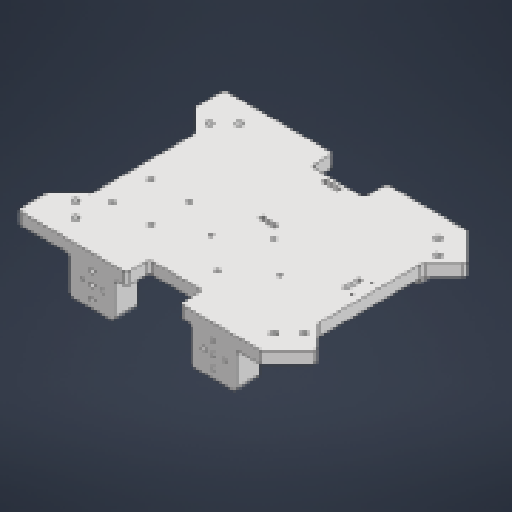
# Autodesk Inventor part: electronics panel
Saved by Autodesk Inventor 2023 (Build 270158000, 158)
## iProperties
Created: 2023-01-16
Part Number: electronics panel
Material: Generic
Document SubType Name: Modeling
Designer: Michael
Density: 1 g/cm^3
Appearance: Default
Author: Michael
Autodesk Inventor part; units mm, degrees
ref_plane "YZ Plane" through (0, 0, 0) normal (1, 0, 0) x (0, 1, 0)
ref_plane "XZ Plane" through (0, 0, 0) normal (0, 1, 0) x (-1, 0, 0)
ref_plane "XY Plane" through (0, 0, 0) normal (0, 0, 1) x (1, 0, 0)
sketch "Sketch2" plane through (0, 0, 0) normal (0, 1, 0) x (-1, 0, 0)
  line L0 (0, 0) -> (177.8, 0)
  line L1 (177.8, 0) -> (177.8, -127)
  line L2 (177.8, -127) -> (0, -127)
  line L3 (0, -127) -> (0, 0)
  line L4 (155.3506, 0) -> (177.8, -22.4519) projected
  line L5 (177.8, -104.5481) -> (155.3506, -127) projected
  line L6 (0, -22.4519) -> (22.4494, 0) projected
  line L7 (22.4494, -127) -> (0, -104.5481) projected
  line L8 (155.3506, 0) -> (173.3121, 17.9595)
  line L9 (173.3121, 17.9595) -> (195.7615, -4.4923)
  line L10 (195.7615, -4.4923) -> (177.8, -22.4519)
  line L11 (177.8, -63.5) -> (0, -63.5)
  line L12 (88.9, -127) -> (88.9, 0)
  line L13 (155.3506, -127) -> (177.8, -104.5481)
  line L14 (155.3506, -127) -> (173.3121, -144.9595)
  line L15 (173.3121, -144.9595) -> (195.7615, -122.5077)
  line L16 (195.7615, -122.5077) -> (177.8, -104.5481)
  line L17 (22.4494, 0) -> (0, -22.4519)
  line L18 (0, -104.5481) -> (22.4494, -127)
  line L19 (22.4494, 0) -> (4.4879, 17.9595)
  line L20 (4.4879, 17.9595) -> (-17.9615, -4.4923)
  line L21 (-17.9615, -4.4923) -> (0, -22.4519)
  line L22 (4.4879, -144.9595) -> (-17.9615, -122.5077)
  line L23 (22.4494, -127) -> (4.4879, -144.9595)
  line L24 (-17.9615, -122.5077) -> (0, -104.5481)
  line L25 (-17.9615, -122.5077) -> (-17.9615, -144.9595)
  line L26 (-17.9615, -144.9595) -> (4.4879, -144.9595)
  line L27 (173.3121, -144.9595) -> (195.7615, -144.9595)
  line L28 (195.7615, -144.9595) -> (195.7615, -122.5077)
  line L29 (195.7615, -4.4923) -> (195.7615, 17.9595)
  line L30 (195.7615, 17.9595) -> (173.3121, 17.9595)
  line L31 (-17.9615, -4.4923) -> (-17.9615, 17.9595)
  line L32 (4.4879, 17.9595) -> (-17.9615, 17.9595)
  line L33 (4.4879, -144.9595) -> (42.5879, -144.9595)
  line L34 (42.5879, -144.9595) -> (42.5879, -127)
  line L35 (173.3121, -144.9595) -> (135.2121, -144.9595)
  line L36 (135.2121, -144.9595) -> (135.2121, -127)
  line L37 (4.4879, 17.9595) -> (42.5879, 17.9595)
  line L38 (42.5879, 17.9595) -> (42.5879, 0)
  line L39 (173.3121, 17.9595) -> (135.2121, 17.9595)
  line L40 (135.2121, 17.9595) -> (135.2121, 0)
  circle A0 centre (178.6987, -10.7776) radius 2.4765 projected
  circle A1 centre (167.025, 0.8974) radius 2.4765 projected
  circle A2 centre (10.775, 0.8974) radius 2.4765 projected
  circle A3 centre (-0.8987, -10.7776) radius 2.4765 projected
  circle A4 centre (10.775, -127.8974) radius 2.4765 projected
  circle A5 centre (-0.8987, -116.2224) radius 2.4765 projected
  circle A6 centre (178.6987, -116.2224) radius 2.4765 projected
  circle A7 centre (167.025, -127.8974) radius 2.4765 projected
  dimension "d0" = 177.8
  dimension "d1" = 127
  dimension "d30" = 25.4
  dimension "d80" = 38.1
  constraints: 74 end point, 12 symmetric about line, 8 perpendicular, 5 point on line, 4 midpoint, 2 horizontal, 2 parallel
  measures "d0" distance of L1.end L2.end
  measures "d1" distance of L0.end L1.end
  measures "d30" distance of L4.start L8.end
  measures "d80" distance of L23.end L33.end
extrude "Extrusion8" add sketch "Sketch2" against normal blind 9.525 contours L19 L37 L38 L0 | L6 L3 A3 L0 A2 | L0 L12 L11 L3 L6 | L0 A2 L3 A3 L21 L20 L19 | L0 L4 L1 L11 L12 | L11 L12 L2 L7 L3 | L40 L39 L8 L0 | L11 L1 L5 L2 L12 | L7 L2 A4 L3 A5 | L3 A5 L2 A4 L23 L22 L24 | L8 L9 L10 L1 A0 L0 A1 | L0 A1 L1 A0 L4 | L2 L34 L33 L23 | L30 L29 L9 | L16 L15 L14 L2 A7 L1 A6 | L1 A6 L2 A7 L5 | L2 L14 L35 L36 | L28 L27 L15
sketch "Sketch8" plane through (0, 0, 0) normal (0, 1, 0) x (1, 0, 0)
  line L0 (-42.5879, 127) -> (-135.2121, 127) projected
  line L1 (0, 22.4519) -> (0, 104.5481) projected
  line L2 (-135.2121, 0) -> (-42.5879, 0) projected
  line L3 (-177.8, 104.5481) -> (-177.8, 22.4519) projected
  line L4 (-145.2802, 116.9307) -> (-173.3121, 144.9595) projected
  line L5 (-195.7615, 122.5077) -> (-177.8, 104.5481) projected
  line L6 (-177.8, 22.4519) -> (-195.7615, 4.4923) projected
  line L7 (-173.3121, -17.9595) -> (-145.2802, 10.0693) projected
  line L8 (-32.5198, 10.0693) -> (-4.4879, -17.9595) projected
  line L9 (17.9615, 4.4923) -> (0, 22.4519) projected
  line L10 (0, 104.5481) -> (17.9615, 122.5077) projected
  line L11 (-4.4879, 144.9595) -> (-32.5198, 116.9307) projected
  line L12 (-135.2121, 127) -> (-129.9506, 127)
  line L13 (-173.3121, 144.9595) -> (-135.2121, 144.9595)
  line L14 (-135.2121, 144.9595) -> (-135.2121, 127)
  line L15 (-42.5879, 127) -> (-135.2121, 127) projected
  line L16 (-135.2121, 127) -> (-109.8121, 127)
  line L17 (-109.8121, 127) -> (-109.8121, 144.9595)
  line L18 (-109.8121, 144.9595) -> (-135.2121, 144.9595)
  line L19 (-135.2121, 144.9595) -> (-135.2121, 127)
  line L20 (-42.5879, 0) -> (-135.2121, 0) projected
  line L21 (-88.9, 0) -> (-88.9, 127)
  line L22 (0, 104.5481) -> (0, 22.4519) projected
  line L23 (0, 63.5) -> (-177.8, 63.5)
  line L24 (-135.2121, 0) -> (-173.3121, -17.9595)
  line L25 (-135.2121, 0) -> (-129.9506, 0)
  line L26 (-173.3121, -17.9595) -> (-135.2121, -17.9595)
  line L27 (-135.2121, -17.9595) -> (-135.2121, 0)
  line L28 (-135.2121, 0) -> (-109.8121, 0)
  line L29 (-109.8121, 0) -> (-109.8121, -17.9595)
  line L30 (-109.8121, -17.9595) -> (-135.2121, -17.9595)
  line L31 (-135.2121, -17.9595) -> (-135.2121, 0)
  line L32 (-42.5879, 0) -> (-135.2121, 0)
  line L33 (-42.5879, 127) -> (-4.4879, 144.9595)
  line L34 (-4.4879, -17.9595) -> (-42.5879, 0)
  line L35 (-42.5879, 127) -> (-47.8494, 127)
  line L36 (-4.4879, 144.9595) -> (-42.5879, 144.9595)
  line L37 (-42.5879, 144.9595) -> (-42.5879, 127)
  line L38 (-67.9879, 127) -> (-67.9879, 144.9595)
  line L39 (-67.9879, 144.9595) -> (-42.5879, 144.9595)
  line L40 (-42.5879, 0) -> (-47.8494, 0)
  line L41 (-67.9879, 0) -> (-67.9879, -17.9595)
  line L42 (-42.5879, -17.9595) -> (-42.5879, 0)
  line L43 (-67.9879, -17.9595) -> (-42.5879, -17.9595)
  line L44 (-4.4879, -17.9595) -> (-42.5879, -17.9595)
  point P0 (0, 0)
  point P1 (-109.8121, 127)
  point P2 (-109.8121, 0)
  point P3 (-22.4494, -17.9595)
  point P4 (-67.9879, 0)
  point P5 (-22.4494, 144.9595)
  point P6 (-67.9879, 127)
  dimension "d54" = 25.4
  dimension "d56" = 0
  constraints: 60 end point, 17 symmetric about line, 4 midpoint, 3 horizontal, 2 parallel, 2 perpendicular
  measures "d54" distance of L18.end L17.end
  measures "d56" distance between parallel lines of L18 L13
extrude "Extrusion10" add sketch "Sketch8" against normal blind 9.525
sketch "Sketch10" plane through (0, -9.525, 0) normal (0, -1, 0) x (1, 0, 0)
  line L0 (-23.5379, -144.9595) -> (-23.5379, -127)
  line L1 (-109.8121, -127) -> (-67.9879, -127) projected
  line L2 (-67.9879, 0) -> (-109.8121, 0) projected
  line L3 (0, -104.5481) -> (0, -22.4519) projected
  line L4 (-177.8, -22.4519) -> (-177.8, -104.5481) projected
  line L5 (0, -63.5) -> (-177.8, -63.5)
  line L6 (-177.8, -104.5481) -> (-177.8, -22.4519) projected
  line L7 (-67.9879, -127) -> (-109.8121, -127) projected
  line L8 (-88.9, -127) -> (-88.9, 0)
  line L9 (-23.5379, -127) -> (-58.4629, -127)
  line L10 (-58.4629, -127) -> (-58.4629, -144.9595)
  line L11 (-58.4629, -144.9595) -> (-23.5379, -144.9595)
  line L12 (-23.5379, -144.9595) -> (-23.5379, -127)
  line L13 (-154.2621, -127) -> (-119.3371, -127)
  line L14 (-119.3371, -127) -> (-119.3371, -144.9595)
  line L15 (-119.3371, -144.9595) -> (-154.2621, -144.9595)
  line L16 (-154.2621, -144.9595) -> (-154.2621, -127)
  line L17 (-23.5379, 17.9595) -> (-23.5379, 0)
  line L18 (-23.5379, 0) -> (-58.4629, 0)
  line L19 (-58.4629, 0) -> (-58.4629, 17.9595)
  line L20 (-58.4629, 17.9595) -> (-23.5379, 17.9595)
  line L21 (-119.3371, 0) -> (-119.3371, 17.9595)
  line L22 (-154.2621, 0) -> (-119.3371, 0)
  line L23 (-154.2621, 17.9595) -> (-154.2621, 0)
  line L24 (-119.3371, 17.9595) -> (-154.2621, 17.9595)
  point P0 (0, 0)
  point P1 (-67.9879, -144.9595)
  point P2 (-109.8121, -144.9595)
  point P3 (-42.5879, -127)
  point P4 (-135.2121, -127)
  point P5 (-42.5879, 0)
  point P6 (-135.2121, 0)
  dimension "d81" = 34.925
  constraints: 38 end point, 14 symmetric about line, 4 midpoint, 2 parallel, 1 horizontal, 1 perpendicular
  measures "d81" distance of L11.end L10.end
extrude "Extrusion11" add sketch "Sketch10" along normal blind 28.575
sketch "Sketch13" plane through (-109.8121, 0, -144.9595) normal (0, 0, -1) x (-1, 0, 0)
  line L0 (34.986, -21.615) -> (18.9865, -21.615)
  line L1 (26.9862, -31.115) -> (26.9862, -12.115)
  line L2 (44.45, -34.925) -> (0, -34.925) projected
  line L3 (0, 0) -> (0, -9.525) projected
  line L4 (-41.8241, -9.525) -> (0, -9.525) projected
  line L5 (-20.9121, -9.525) -> (-20.9121, -25.2345)
  line L6 (-76.8101, -21.615) -> (-60.8106, -21.615)
  line L7 (-68.8104, -31.115) -> (-68.8104, -12.115)
  line L8 (9.525, -9.525) -> (9.525, -38.1) projected
  point P0 (-109.8121, 0)
  point P1 (26.9862, -21.615)
  point P2 (0, -34.925)
  point P3 (-82.1012, -6.35)
  point P4 (-68.8104, -21.615)
  point P5 (-67.2241, -9.525)
  dimension "d66" = 15.9995
  dimension "d67" = 19
  dimension "d68" = 3.81
  dimension "d83" = 9.4615
  constraints: 10 end point, 9 symmetric about line, 8 coincident, 2 midpoint, 2 vertical, 1 horizontal, 3 other
  measures "d66" distance of L0.start L0.end
  measures "d67" distance of L1.start L1.end
  measures "d83" distance from line of L8 L0.end
hole "Hole2" at (-136.7983, -21.615, -144.9595) at (-144.798, -21.615, -144.9595) at (-136.7983, -31.115, -144.9595) at (-128.7986, -21.615, -144.9595) at (-136.7983, -12.115, -144.9595) at (-41.0017, -12.115, -144.9595) at (-49.0014, -21.615, -144.9595) at (-41.0017, -31.115, -144.9595) at (-33.002, -21.615, -144.9595) at (-41.0017, -21.615, -144.9595) direction (0, 0, 1) diameter 3.3985 end through all
fillet "Fillet1" radius 2.54 28 edges at (-23.5379, -9.525, -135.9798) (-58.4629, -9.525, -135.9798) (-58.4629, -9.525, 8.9798) (-23.5379, -9.525, 8.9798) (-119.3371, -9.525, -135.9798) (-119.3371, -9.525, 8.9798) (-119.3371, -38.1, 8.9798) (-23.5379, -38.1, 8.9798) (-23.5379, -38.1, -135.9798) (-119.3371, -38.1, -135.9798) (-58.4629, -38.1, -135.9798) (-154.2621, -38.1, -135.9798) (-58.4629, -38.1, 8.9798) (-154.2621, -38.1, 8.9798) (-154.2621, -9.525, 8.9798) (-154.2621, -9.525, -135.9798) (-67.9879, -4.7625, 17.9595) (-109.8121, -4.7625, 17.9595) (-195.7615, -4.7625, 17.9595) (-67.9879, -4.7625, -144.9595) (-195.7615, -4.7625, -144.9595) (-109.8121, -4.7625, -144.9595) (-67.9879, -4.7625, -127) (-109.8121, -4.7625, -127) (-109.8121, -4.7625, 0) (-67.9879, -4.7625, 0) (-195.7615, -4.7625, -4.4923) (-195.7615, -4.7625, -122.5077)
fillet "Fillet2" radius 3.175 6 edges at (-177.8, -4.7625, -104.5481) (-177.8, -4.7625, -22.4519) (0, -4.7625, -104.5481) (0, -4.7625, -22.4519) (17.9615, -4.7625, -4.4923) (17.9615, -4.7625, -122.5077)
sketch "Sketch14" plane through (0, 0, 0) normal (0, 1, 0) x (1, 0, 0)
  line L0 (0, 23.7671) -> (0, 103.2329) projected
  line L1 (0, 103.2329) -> (0, 23.7671) projected
  line L2 (0, 63.5) -> (-12.6589, 63.5)
  line L3 (0, 23.7671) -> (-12.6589, 23.7671)
  arc A0 (0.9301, 105.4781) -> (0, 103.2329) centre (3.175, 103.2329) ccw projected
  line L4 (0, 103.2329) -> (-12.6589, 103.2329)
  point P0 (0, 0)
  point P1 (-6.3246, 55.5625)
  point P2 (-6.3295, 63.5)
  point P3 (-6.3246, 71.4375)
  dimension "d89" = 7.9375
  dimension "d90" = 6.3246
  constraints: 6 end point, 3 horizontal, 2 midpoint, 1 symmetric about line
  measures "d89" distance of point (-6.329, 63.5) point (-6.325, 55.563)
  measures "d90" distance from line of L0 point (-6.325, 55.563)
hole "Hole3" at (-6.3246, 0, -55.5625) at (-6.3246, 0, -71.4375) direction (0, -1, 0) diameter 1.5999 end through all
sketch "Sketch16" plane through (0, 0, 0) normal (0, 1, 0) x (1, 0, 0)
  point P0 (0, 0)
  point P1 (-163.5597, 24.5234)
  point P2 (-163.9076, 55.0214)
  point P3 (-133.4076, 55.0736)
  point P4 (-133.0597, 24.5756)
  dimension "d109" = 30.5
  dimension "d110" = 30.5
  dimension "d111" = 30.5
  dimension "d112" = 30.5
  constraints: 1 other
  measures "d109" distance of point (-163.908, 55.021) point (-163.56, 24.523)
  measures "d110" distance of point (-133.408, 55.074) point (-133.06, 24.576)
  measures "d111" distance of point (-133.06, 24.576) point (-163.56, 24.523)
  measures "d112" distance of point (-133.408, 55.074) point (-163.908, 55.021)
hole "Hole5" at (-163.5597, 0, -24.5234) at (-163.9076, 0, -55.0214) at (-133.4076, 0, -55.0736) at (-133.0597, 0, -24.5756) direction (0, -1, 0) diameter 4 end through all
sketch "Sketch17" plane through (0, 0, 0) normal (0, 1, 0) x (1, 0, 0)
  line L0 (-127.2393, 115.3557) -> (-127.2393, 74.7157) projected
  line L1 (-127.2393, 74.7157) -> (-51.0393, 74.7157) projected
  line L2 (-51.0393, 74.7157) -> (-51.0393, 115.3557) projected
  line L3 (-51.0393, 115.3557) -> (-127.2393, 115.3557) projected
  line L4 (-70.5279, 127) -> (-107.2721, 127) projected
  line L5 (-107.2721, 127) -> (-70.5279, 127) projected
  line L6 (-88.9, 127) -> (-88.9, 71.6642)
  line L7 (-88.9, 120.839) -> (-95.25, 120.839)
  line L8 (-95.25, 120.839) -> (-95.25, 124.014)
  line L9 (-95.25, 124.014) -> (-88.9, 124.014)
  line L10 (-88.9, 124.014) -> (-88.9, 120.839)
  line L11 (-88.9, 120.839) -> (-82.55, 120.839)
  line L12 (-82.55, 120.839) -> (-82.55, 124.014)
  line L13 (-82.55, 124.014) -> (-88.9, 124.014)
  line L14 (-88.9, 124.014) -> (-88.9, 120.839)
  line L15 (-88.9, 71.0389) -> (-95.25, 71.0389)
  line L16 (-95.25, 71.0389) -> (-95.25, 74.2139)
  line L17 (-95.25, 74.2139) -> (-88.9, 74.2139)
  line L18 (-88.9, 74.2139) -> (-88.9, 71.0389)
  line L19 (-88.9, 71.0389) -> (-82.55, 71.0389)
  line L20 (-82.55, 71.0389) -> (-82.55, 74.2139)
  line L21 (-82.55, 74.2139) -> (-88.9, 74.2139)
  line L22 (-88.9, 74.2139) -> (-88.9, 71.0389)
  point P0 (0, 0)
  point P1 (-87.3125, 128.5875)
  dimension "d120" = 6.35
  dimension "d121" = 3.175
  dimension "d122" = 6.35
  dimension "d123" = 6.35
  dimension "d124" = 3.175
  dimension "d125" = 6.35
  constraints: 34 end point, 8 parallel, 5 perpendicular, 4 horizontal, 4 point on line, 1 midpoint
  measures "d120" distance of L8.end L9.end
  measures "d121" distance of L7.end L8.end
  measures "d122" distance of L13.end L12.end
  measures "d123" distance of L16.end L18.start
  measures "d124" distance of L15.end L16.end
  measures "d125" distance of L21.end L21.start
extrude "Extrusion14" cut sketch "Sketch17" against normal blind 11.1125 contours L13 L12 L11 L6 | L6 L7 L8 L9 | L21 L20 L19 L18 L6 | L6 L18 L15 L16 L17
sketch "Sketch18" plane through (0, 0, 0) normal (0, 1, 0) x (1, 0, 0)
  circle A0 centre (-75.1754, 63.026) radius 1.6 projected
  circle A1 centre (-102.2121, 41.0261) radius 1.6 projected
  circle A2 centre (-75.1754, 19.0261) radius 1.6076 projected
  circle A3 centre (-48.2121, 41.0261) radius 1.6 projected
  point P0 (0, 0)
extrude "Extrusion15" cut sketch "Sketch18" against normal blind 14.2875
sketch "Sketch19" plane through (0, 0, 0) normal (0, 1, 0) x (1, 0, 0)
  line L0 (-14.8408, 57.15) -> (-11.6658, 57.15)
  line L1 (-11.6658, 57.15) -> (-11.6658, 69.85)
  line L2 (-11.6658, 69.85) -> (-14.8408, 69.85)
  line L3 (-14.8408, 69.85) -> (-14.8408, 57.15)
  circle A0 centre (-6.3246, 55.5625) radius 0.8 projected
  circle A1 centre (-6.3246, 71.4375) radius 0.8 projected
  line L4 (-6.3246, 55.5625) -> (-14.8408, 55.5625)
  circle A2 centre (-6.3246, 71.4375) radius 0.8 projected
  line L5 (-6.3246, 71.4375) -> (-14.8408, 71.4375)
  point P0 (0, 0)
  point P1 (-13.2533, 57.15)
  dimension "d130" = 3.175
  dimension "d131" = 12.7
  dimension "d132" = 1.5875
  constraints: 12 end point, 3 horizontal, 2 parallel, 1 midpoint, 1 perpendicular
  measures "d130" distance of L2.end L1.end
  measures "d131" distance of L1.end L0.end
  measures "d132" distance from line of L4 point (-13.253, 57.15)
extrude "Extrusion16" cut sketch "Sketch19" against normal blind 25.4 contours L3 L2 L1 L0
body "Solid3"
